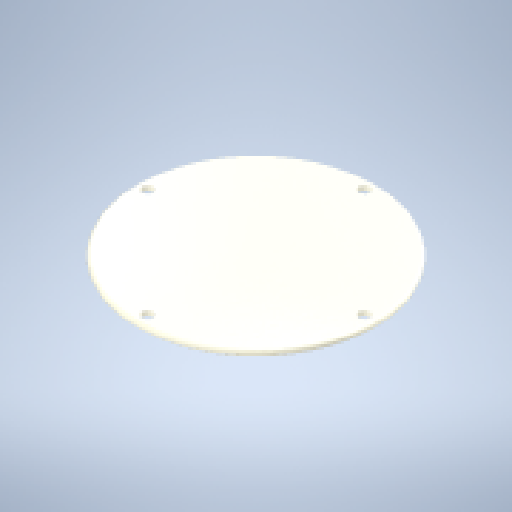
# Autodesk Inventor part: Base_Cover
Saved by Autodesk Inventor 2025.3 (Build 293356000, 356)
## iProperties
Created: 2026-01-15
Part Number: Base_Cover
Material: Acetal Resin, White
Document SubType Name: Modeling
Designer: Balint
Density: 1.425 g/cm^3
Appearance: Smooth - White
Author: Balint
Autodesk Inventor part; units mm, degrees
ref_plane "YZ Plane" through (0, 0, 0) normal (1, 0, 0) x (0, 1, 0)
ref_plane "XZ Plane" through (0, 0, 0) normal (0, 1, 0) x (-1, 0, 0)
ref_plane "XY Plane" through (0, 0, 0) normal (0, 0, 1) x (1, 0, 0)
sketch "Sketch4" plane through (0, 0, 0) normal (0, 1, 0) x (-1, 0, 0)
  circle A0 centre (-1.9122, 1.2943) radius 36.25 projected
  circle A1 centre (0, 0) radius 45.5
  circle A2 centre (41.25, 0) radius 2.05
  circle A3 centre (0, 41.25) radius 2.05
  circle A4 centre (-41.25, 0) radius 2.05
  circle A5 centre (0, -41.25) radius 2.05
  dimension "d18" = 91
  dimension "d20" = 4.1
  dimension "d23" = 360
  constraints: 5 centre point, 1 coincident, 9 other
  measures "d18" diameter of A1
  measures "d20" diameter of A2
extrude "Extrusion4" add sketch "Sketch4" along normal blind 2.5 contours A0 | A1
sketch "Sketch5" plane through (0, 0, 0) normal (0, -1, 0) x (1, 0, 0)
  circle A0 centre (-41.25, 0) radius 2.05 projected
  circle A1 centre (0, 41.25) radius 2.05 projected
  circle A2 centre (41.25, 0) radius 2.05 projected
  circle A3 centre (0, -41.25) radius 2.05 projected
  circle A4 centre (-41.25, 0) radius 3
  circle A5 centre (0, 41.25) radius 3
  circle A6 centre (41.25, 0) radius 3
  circle A7 centre (0, -41.25) radius 3
  point P0 (0, 0)
  dimension "d27" = 6
  dimension "d28" = 6
  dimension "d29" = 6
  dimension "d30" = 6
  constraints: 4 centre point, 4 coincident
  measures "d27" diameter of A4
  measures "d28" diameter of A5
  measures "d29" diameter of A6
  measures "d30" diameter of A7
extrude "Extrusion5" cut sketch "Sketch5" against normal blind 1.25 contours A0 | A1 | A2 | A3 | A4 | A5 | A6 | A7
fillet "Fillet2" radius 1 2 edges at (45.5, 0, 0) (45.5, 2.5, 0)
body "Solid2"
